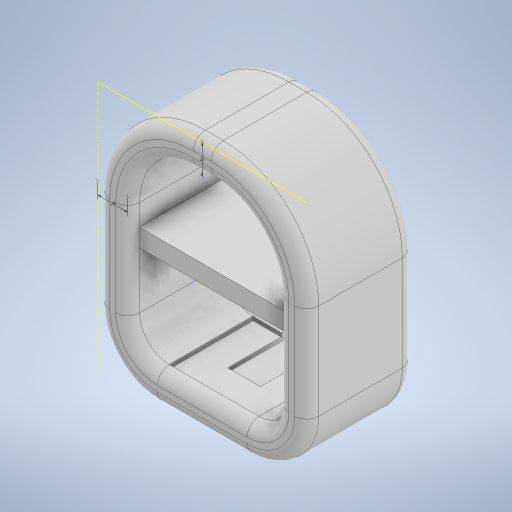
# Autodesk Inventor part: headset_charger333344
Saved by Autodesk Inventor 2024 (Build 280153000, 153)
## iProperties
Created: 2024-09-09
Part Number: headset_charger333344
Material: 일반
Document SubType Name: Modeling
Designer: ghkdc
Density: 1 g/cm^3
Appearance: 기본값
Author: ghkdc
Autodesk Inventor part; units mm, degrees
ref_plane "YZ Plane" through (0, 0, 0) normal (1, 0, 0) x (0, 1, 0)
ref_plane "XZ Plane" through (0, 0, 0) normal (0, 1, 0) x (-1, 0, 0)
ref_plane "XY Plane" through (0, 0, 0) normal (0, 0, 1) x (1, 0, 0)
sketch "스케치1" plane through (0, 0, 0) normal (0, 0, 1) x (1, 0, 0)
  line L0 (87.5, -105) -> (-87.5, -105)
  line L1 (-87.5, -105) -> (-87.5, 105)
  line L2 (-87.5, 105) -> (87.5, 105)
  line L3 (87.5, 105) -> (87.5, -105)
  line L4 (87.5, -105) -> (-87.5, 105) construction
  line L5 (-87.5, -105) -> (87.5, 105) construction
  point P0 (0, 0)
  dimension "d0" = 210
  dimension "d1" = 175
  constraints: 12 end point, 2 midpoint, 2 parallel, 1 horizontal, 1 perpendicular
  measures "d0" distance of L0.end L1.end
  measures "d1" distance of L1.end L2.end
extrude "돌출1" add sketch "스케치1" along normal blind 90
sketch "스케치2" plane through (0, 0, 90) normal (0, 0, 1) x (1, 0, 0)
  line L0 (87.5, 105) -> (-87.5, 105) projected
  line L1 (-87.5, 105) -> (-87.5, -105) projected
  point P0 (0, 0)
  point P1 (0, 80)
  point P2 (0, 105)
  point P3 (-87.5, 34.2904)
  point P4 (-62.5, 34.2904)
  dimension "d4" = 25
  dimension "d5" = 25
  constraints: 1 midpoint, 1 point on line
  measures "d4" distance of point (0, 80) point (0, 105)
  measures "d5" distance of point (-62.5, 34.29) point (-87.5, 34.29)
sketch "스케치3" plane through (0, 0, 90) normal (0, 0, 1) x (1, 0, 0)
  point P0 (0, 0)
fillet "모깎기3" radius 80 2 edges at (-87.5, 105, 45) (87.5, 105, 45)
fillet "모깎기4" radius 50 2 edges at (-87.5, -105, 45) (87.5, -105, 45)
shell "쉘1" thickness 25 removed faces 2 at (-29.1667, -28.3333, 90) at (-29.1667, -28.3333, 0)
fillet "모깎기5" radius 10 14 edges at (46.3909, 63.8909, 90) (62.5, -15, 90) (55.1777, -72.6777, 90) (0, 80, 90) (-46.3909, 63.8909, 90) (-62.5, -15, 90) (-55.1777, -72.6777, 90) (0, 80, 0) (-46.3909, 63.8909, 0) (-62.5, -15, 0) (-55.1777, -72.6777, 0) (62.5, -15, 0) (55.1777, -72.6777, 0) (46.3909, 63.8909, 0)
fillet "모깎기6" radius 10 16 edges at (64.0685, 81.5685, 0) (0, 105, 0) (-64.0685, 81.5685, 0) (-87.5, -15, 0) (-72.8553, -90.3553, 0) (0, -105, 0) (72.8553, -90.3553, 0) (87.5, -15, 0) (87.5, -15, 90) (72.8553, -90.3553, 90) (0, -105, 90) (-72.8553, -90.3553, 90) (-87.5, -15, 90) (-64.0685, 81.5685, 90) (0, 105, 90) (64.0685, 81.5685, 90)
sketch "스케치7" plane through (-37.5, -80, 10) normal (0, 1, 0) x (1, 0, 0)
  line L0 (0, -80) -> (0, -70) projected
  line L1 (0, -70) -> (74.9762, -70)
  line L2 (74.9762, -70) -> (74.9762, -0.0201)
  line L3 (74.9762, -0.0201) -> (0, -0.0201)
  line L4 (0, -0.0201) -> (0, -70)
  point P0 (37.5, 10)
  constraints: 8 end point, 2 parallel, 1 horizontal, 1 perpendicular
extrude "돌출5" cut sketch "스케치7" against normal blind 3
sketch "스케치8" plane through (-37.5, -83, 10) normal (0, 1, 0) x (1, 0, 0)
  point P0 (37.5, 10)
sketch "스케치9" plane through (62.5, -55, 10) normal (-1, 0, 0) x (0, 0, 1)
  line L0 (0, 0) -> (0, 80) projected
  line L1 (70, 80) -> (70, 0) projected
  line L2 (0, 62.1326) -> (70, 62.1326)
  line L3 (70, 62.1326) -> (70, 47.1326)
  line L4 (70, 47.1326) -> (0, 47.1326)
  line L5 (0, 47.1326) -> (0, 62.1326)
  point P0 (-10, 55)
  point P1 (0, 47.1326)
  dimension "d24" = 15
  constraints: 8 end point, 2 parallel, 2 point on line, 1 horizontal, 1 perpendicular
  measures "d24" distance between parallel lines of L4 L2
extrude "돌출6" add sketch "스케치9" along normal up to surface (125 mm away)
sketch "스케치10" plane through (-37.5, -83, 10) normal (0, 1, 0) x (1, 0, 0)
  point P0 (37.5, 10)
sketch "스케치11" plane through (-37.5, -83, 10) normal (0, 1, 0) x (1, 0, 0)
  line L0 (23.9, 53.6654) -> (51.1, 53.6654)
  line L1 (51.1, 53.6654) -> (51.1, -44.9021)
  line L2 (51.1, -44.9021) -> (23.9, -44.9021)
  line L3 (23.9, -44.9021) -> (23.9, 53.6654)
  line L4 (23.9, 53.6654) -> (51.1, -44.9021) construction
  line L5 (51.1, 53.6654) -> (23.9, -44.9021) construction
  point P0 (37.5, 10)
  point P1 (37.5, 4.3816)
  dimension "d25" = 27.2
  constraints: 12 end point, 2 midpoint, 2 parallel, 1 horizontal, 1 perpendicular
  measures "d25" distance of L1.end L2.end
extrude "돌출7" cut sketch "스케치11" against normal blind 3
sketch "스케치12" plane through (-37.5, -80, 10) normal (0, 1, 0) x (1, 0, 0)
  line L0 (0, -0.0201) -> (23.9, -0.0201) projected
  line L1 (51.1, 7.1414) -> (23.9, 7.1414) projected
  line L2 (23.9, -0.0201) -> (51.1, -0.0201)
  line L3 (51.1, -0.0201) -> (51.1, 7.1414)
  line L4 (51.1, 7.1414) -> (23.9, 7.1414)
  line L5 (23.9, 7.1414) -> (23.9, -0.0201)
  point P0 (37.5, 10)
  constraints: 8 end point, 2 parallel, 1 horizontal, 1 perpendicular
extrude "돌출8" cut sketch "스케치12" against normal blind 3
